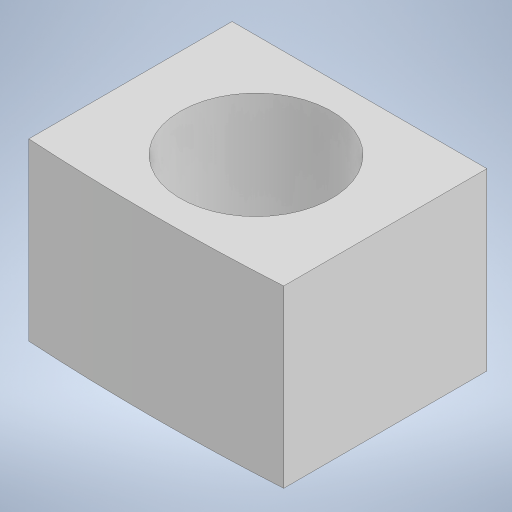
# Autodesk Inventor part: 170x109MagnetHolder
Saved by Autodesk Inventor 2024 (Build 280153000, 153)
## iProperties
Created: 2023-09-22
Part Number: 170x109MagnetHolder
Material: Generic
Document SubType Name: Modeling
Designer: Chris
Density: 1 g/cm^3
Appearance: Default
Author: Chris
Autodesk Inventor part; units mm, degrees
ref_plane "YZ Plane" through (0, 0, 0) normal (1, 0, 0) x (0, 1, 0)
ref_plane "XZ Plane" through (0, 0, 0) normal (0, 1, 0) x (-1, 0, 0)
ref_plane "XY Plane" through (0, 0, 0) normal (0, 0, 1) x (1, 0, 0)
sketch "Sketch1" plane through (0, 0, 0) normal (0, 1, 0) x (-1, 0, 0)
  ellipse E0 centre (0, 0) end of major axis (0, -170) minor radius 109
  ellipse E1 centre (0, 0) end of major axis (105.5, 0) minor radius 166.5
  line L0 (29.1902, 160) -> (-29.1902, 160)
  circle A0 centre (0, 163.25) radius 2.375
  line L1 (4, 166.3803) -> (4, 160)
  line L2 (-4, 166.3803) -> (-4, 160)
  line L3 (0, 170) -> (0, 0)
  point P0 (-4, 163.1901)
  dimension "d0" = 170
  dimension "d1" = 109
  dimension "d2" = 105.5
  dimension "d3" = 166.5
  dimension "d4" = 160
  dimension "d5" = 4.75
  dimension "d6" = 3.25
  dimension "d7" = 4
  dimension "d8" = 4
  dimension "d9" = 163.25
  constraints: 8 end point, 2 coincident, 2 perpendicular, 2 point on line, 1 centre point, 1 horizontal, 1 midpoint, 1 vertical, 1 vertical alignment, 8 other
  measures "d4" distance from line of L3.end L0
  measures "d5" diameter of A0
  measures "d6" distance from line of L0 A0.centre
  measures "d7" distance from line of L1 A0.centre
  measures "d8" horizontal distance of point (-4, 163.19) A0.centre
  measures "d9" distance of point (0, 0) A0.centre
extrude "Extrusion1" add sketch "Sketch1" along normal blind 5.5 contours L3 A0 L0 L2 E1 | E1 L1 L0 L3 A0
body "Solid1"
